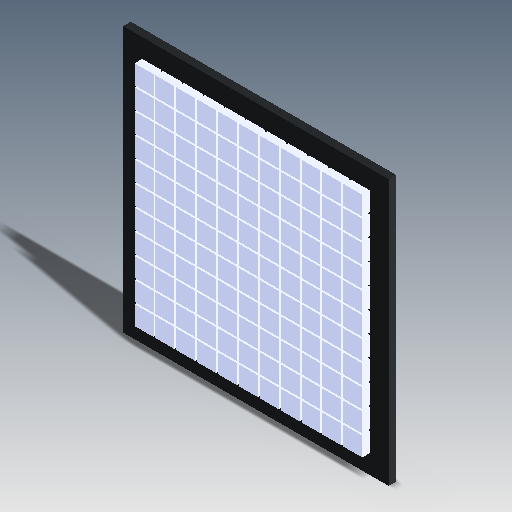
# Autodesk Inventor part: Phase Meter
Saved by Autodesk Inventor 2026 (Build 300175050, 175E)
## iProperties
Created: 2025-08-02
Part Number: Phase Meter
Material: Generic
Document SubType Name: Modeling
Designer: aman0
Density: 1 g/cm^3
Appearance: Default
Author: aman0
Autodesk Inventor part; units mm, degrees
ref_plane "YZ Plane" through (0, 0, 0) normal (1, 0, 0) x (0, 1, 0)
ref_plane "XZ Plane" through (0, 0, 0) normal (0, 1, 0) x (-1, 0, 0)
ref_plane "XY Plane" through (0, 0, 0) normal (0, 0, 1) x (1, 0, 0)
sketch "Sketch1" plane through (0, 0, 0) normal (0, 0, 1) x (1, 0, 0)
  line L0 (-1.25, -1.25) -> (1.25, -1.25)
  line L1 (1.25, -1.25) -> (1.25, 1.25)
  line L2 (1.25, 1.25) -> (-1.25, 1.25)
  line L3 (-1.25, 1.25) -> (-1.25, -1.25)
  line L4 (-1.25, -1.25) -> (1.25, 1.25) construction
  line L5 (1.25, -1.25) -> (-1.25, 1.25) construction
  line L6 (-4, -1.25) -> (-1.5, -1.25)
  line L7 (-1.5, -1.25) -> (-1.5, 1.25)
  line L8 (-1.5, 1.25) -> (-4, 1.25)
  line L9 (-4, 1.25) -> (-4, -1.25)
  line L10 (-4, -1.25) -> (-1.5, 1.25) construction
  line L11 (-1.5, -1.25) -> (-4, 1.25) construction
  line L12 (1.5, -1.25) -> (4, -1.25)
  line L13 (4, -1.25) -> (4, 1.25)
  line L14 (4, 1.25) -> (1.5, 1.25)
  line L15 (1.5, 1.25) -> (1.5, -1.25)
  line L16 (1.5, -1.25) -> (4, 1.25) construction
  line L17 (4, -1.25) -> (1.5, 1.25) construction
  line L18 (-6.75, -1.25) -> (-4.25, -1.25)
  line L19 (-4.25, -1.25) -> (-4.25, 1.25)
  line L20 (-4.25, 1.25) -> (-6.75, 1.25)
  line L21 (-6.75, 1.25) -> (-6.75, -1.25)
  line L22 (-6.75, -1.25) -> (-4.25, 1.25) construction
  line L23 (-4.25, -1.25) -> (-6.75, 1.25) construction
  line L24 (4.25, -1.25) -> (6.75, -1.25)
  line L25 (6.75, -1.25) -> (6.75, 1.25)
  line L26 (6.75, 1.25) -> (4.25, 1.25)
  line L27 (4.25, 1.25) -> (4.25, -1.25)
  line L28 (4.25, -1.25) -> (6.75, 1.25) construction
  line L29 (6.75, -1.25) -> (4.25, 1.25) construction
  line L30 (-9.5, -1.25) -> (-7, -1.25)
  line L31 (-7, -1.25) -> (-7, 1.25)
  line L32 (-7, 1.25) -> (-9.5, 1.25)
  line L33 (-9.5, 1.25) -> (-9.5, -1.25)
  line L34 (-9.5, -1.25) -> (-7, 1.25) construction
  line L35 (-7, -1.25) -> (-9.5, 1.25) construction
  line L36 (7, -1.25) -> (9.5, -1.25)
  line L37 (9.5, -1.25) -> (9.5, 1.25)
  line L38 (9.5, 1.25) -> (7, 1.25)
  line L39 (7, 1.25) -> (7, -1.25)
  line L40 (7, -1.25) -> (9.5, 1.25) construction
  line L41 (9.5, -1.25) -> (7, 1.25) construction
  line L42 (-12.25, -1.25) -> (-9.75, -1.25)
  line L43 (-9.75, -1.25) -> (-9.75, 1.25)
  line L44 (-9.75, 1.25) -> (-12.25, 1.25)
  line L45 (-12.25, 1.25) -> (-12.25, -1.25)
  line L46 (-12.25, -1.25) -> (-9.75, 1.25) construction
  line L47 (-9.75, -1.25) -> (-12.25, 1.25) construction
  line L48 (9.75, -1.25) -> (12.25, -1.25)
  line L49 (12.25, -1.25) -> (12.25, 1.25)
  line L50 (12.25, 1.25) -> (9.75, 1.25)
  line L51 (9.75, 1.25) -> (9.75, -1.25)
  line L52 (9.75, -1.25) -> (12.25, 1.25) construction
  line L53 (12.25, -1.25) -> (9.75, 1.25) construction
  line L54 (-15, -1.25) -> (-12.5, -1.25)
  line L55 (-12.5, -1.25) -> (-12.5, 1.25)
  line L56 (-12.5, 1.25) -> (-15, 1.25)
  line L57 (-15, 1.25) -> (-15, -1.25)
  line L58 (-15, -1.25) -> (-12.5, 1.25) construction
  line L59 (-12.5, -1.25) -> (-15, 1.25) construction
  line L60 (12.5, -1.25) -> (15, -1.25)
  line L61 (15, -1.25) -> (15, 1.25)
  line L62 (15, 1.25) -> (12.5, 1.25)
  line L63 (12.5, 1.25) -> (12.5, -1.25)
  line L64 (12.5, -1.25) -> (15, 1.25) construction
  line L65 (15, -1.25) -> (12.5, 1.25) construction
  line L66 (-1.25, -4) -> (1.25, -4)
  line L67 (1.25, -4) -> (1.25, -1.5)
  line L68 (1.25, -1.5) -> (-1.25, -1.5)
  line L69 (-1.25, -1.5) -> (-1.25, -4)
  line L70 (-1.25, -4) -> (1.25, -1.5) construction
  line L71 (1.25, -4) -> (-1.25, -1.5) construction
  line L72 (-4, -4) -> (-1.5, -4)
  line L73 (-1.5, -4) -> (-1.5, -1.5)
  line L74 (-1.5, -1.5) -> (-4, -1.5)
  line L75 (-4, -1.5) -> (-4, -4)
  line L76 (-4, -4) -> (-1.5, -1.5) construction
  line L77 (-1.5, -4) -> (-4, -1.5) construction
  line L78 (1.5, -4) -> (4, -4)
  line L79 (4, -4) -> (4, -1.5)
  line L80 (4, -1.5) -> (1.5, -1.5)
  line L81 (1.5, -1.5) -> (1.5, -4)
  line L82 (1.5, -4) -> (4, -1.5) construction
  line L83 (4, -4) -> (1.5, -1.5) construction
  line L84 (-6.75, -4) -> (-4.25, -4)
  line L85 (-4.25, -4) -> (-4.25, -1.5)
  line L86 (-4.25, -1.5) -> (-6.75, -1.5)
  line L87 (-6.75, -1.5) -> (-6.75, -4)
  line L88 (-6.75, -4) -> (-4.25, -1.5) construction
  line L89 (-4.25, -4) -> (-6.75, -1.5) construction
  line L90 (4.25, -4) -> (6.75, -4)
  line L91 (6.75, -4) -> (6.75, -1.5)
  line L92 (6.75, -1.5) -> (4.25, -1.5)
  line L93 (4.25, -1.5) -> (4.25, -4)
  line L94 (4.25, -4) -> (6.75, -1.5) construction
  line L95 (6.75, -4) -> (4.25, -1.5) construction
  line L96 (-9.5, -4) -> (-7, -4)
  line L97 (-7, -4) -> (-7, -1.5)
  line L98 (-7, -1.5) -> (-9.5, -1.5)
  line L99 (-9.5, -1.5) -> (-9.5, -4)
  line L100 (-9.5, -4) -> (-7, -1.5) construction
  line L101 (-7, -4) -> (-9.5, -1.5) construction
  line L102 (7, -4) -> (9.5, -4)
  line L103 (9.5, -4) -> (9.5, -1.5)
  line L104 (9.5, -1.5) -> (7, -1.5)
  line L105 (7, -1.5) -> (7, -4)
  line L106 (7, -4) -> (9.5, -1.5) construction
  line L107 (9.5, -4) -> (7, -1.5) construction
  line L108 (-12.25, -4) -> (-9.75, -4)
  line L109 (-9.75, -4) -> (-9.75, -1.5)
  line L110 (-9.75, -1.5) -> (-12.25, -1.5)
  line L111 (-12.25, -1.5) -> (-12.25, -4)
  line L112 (-12.25, -4) -> (-9.75, -1.5) construction
  line L113 (-9.75, -4) -> (-12.25, -1.5) construction
  line L114 (9.75, -4) -> (12.25, -4)
  line L115 (12.25, -4) -> (12.25, -1.5)
  line L116 (12.25, -1.5) -> (9.75, -1.5)
  line L117 (9.75, -1.5) -> (9.75, -4)
  line L118 (9.75, -4) -> (12.25, -1.5) construction
  line L119 (12.25, -4) -> (9.75, -1.5) construction
  line L120 (-15, -4) -> (-12.5, -4)
  line L121 (-12.5, -4) -> (-12.5, -1.5)
  line L122 (-12.5, -1.5) -> (-15, -1.5)
  line L123 (-15, -1.5) -> (-15, -4)
  line L124 (-15, -4) -> (-12.5, -1.5) construction
  line L125 (-12.5, -4) -> (-15, -1.5) construction
  line L126 (12.5, -4) -> (15, -4)
  line L127 (15, -4) -> (15, -1.5)
  line L128 (15, -1.5) -> (12.5, -1.5)
  line L129 (12.5, -1.5) -> (12.5, -4)
  line L130 (12.5, -4) -> (15, -1.5) construction
  line L131 (15, -4) -> (12.5, -1.5) construction
  line L132 (-1.25, 1.5) -> (1.25, 1.5)
  line L133 (1.25, 1.5) -> (1.25, 4)
  line L134 (1.25, 4) -> (-1.25, 4)
  line L135 (-1.25, 4) -> (-1.25, 1.5)
  line L136 (-1.25, 1.5) -> (1.25, 4) construction
  line L137 (1.25, 1.5) -> (-1.25, 4) construction
  line L138 (-4, 1.5) -> (-1.5, 1.5)
  line L139 (-1.5, 1.5) -> (-1.5, 4)
  line L140 (-1.5, 4) -> (-4, 4)
  line L141 (-4, 4) -> (-4, 1.5)
  line L142 (-4, 1.5) -> (-1.5, 4) construction
  line L143 (-1.5, 1.5) -> (-4, 4) construction
  line L144 (1.5, 1.5) -> (4, 1.5)
  line L145 (4, 1.5) -> (4, 4)
  line L146 (4, 4) -> (1.5, 4)
  line L147 (1.5, 4) -> (1.5, 1.5)
  line L148 (1.5, 1.5) -> (4, 4) construction
  line L149 (4, 1.5) -> (1.5, 4) construction
  line L150 (-6.75, 1.5) -> (-4.25, 1.5)
  line L151 (-4.25, 1.5) -> (-4.25, 4)
  line L152 (-4.25, 4) -> (-6.75, 4)
  line L153 (-6.75, 4) -> (-6.75, 1.5)
  line L154 (-6.75, 1.5) -> (-4.25, 4) construction
  line L155 (-4.25, 1.5) -> (-6.75, 4) construction
  line L156 (4.25, 1.5) -> (6.75, 1.5)
  line L157 (6.75, 1.5) -> (6.75, 4)
  line L158 (6.75, 4) -> (4.25, 4)
  line L159 (4.25, 4) -> (4.25, 1.5)
  line L160 (4.25, 1.5) -> (6.75, 4) construction
  line L161 (6.75, 1.5) -> (4.25, 4) construction
  line L162 (-9.5, 1.5) -> (-7, 1.5)
  line L163 (-7, 1.5) -> (-7, 4)
  line L164 (-7, 4) -> (-9.5, 4)
  line L165 (-9.5, 4) -> (-9.5, 1.5)
  line L166 (-9.5, 1.5) -> (-7, 4) construction
  line L167 (-7, 1.5) -> (-9.5, 4) construction
  line L168 (7, 1.5) -> (9.5, 1.5)
  line L169 (9.5, 1.5) -> (9.5, 4)
  line L170 (9.5, 4) -> (7, 4)
  line L171 (7, 4) -> (7, 1.5)
  line L172 (7, 1.5) -> (9.5, 4) construction
  line L173 (9.5, 1.5) -> (7, 4) construction
  line L174 (-12.25, 1.5) -> (-9.75, 1.5)
  line L175 (-9.75, 1.5) -> (-9.75, 4)
  line L176 (-9.75, 4) -> (-12.25, 4)
  line L177 (-12.25, 4) -> (-12.25, 1.5)
  line L178 (-12.25, 1.5) -> (-9.75, 4) construction
  line L179 (-9.75, 1.5) -> (-12.25, 4) construction
  line L180 (9.75, 1.5) -> (12.25, 1.5)
  line L181 (12.25, 1.5) -> (12.25, 4)
  line L182 (12.25, 4) -> (9.75, 4)
  line L183 (9.75, 4) -> (9.75, 1.5)
  line L184 (9.75, 1.5) -> (12.25, 4) construction
  line L185 (12.25, 1.5) -> (9.75, 4) construction
  line L186 (-15, 1.5) -> (-12.5, 1.5)
  line L187 (-12.5, 1.5) -> (-12.5, 4)
  line L188 (-12.5, 4) -> (-15, 4)
  line L189 (-15, 4) -> (-15, 1.5)
  line L190 (-15, 1.5) -> (-12.5, 4) construction
  line L191 (-12.5, 1.5) -> (-15, 4) construction
  line L192 (12.5, 1.5) -> (15, 1.5)
  line L193 (15, 1.5) -> (15, 4)
  line L194 (15, 4) -> (12.5, 4)
  line L195 (12.5, 4) -> (12.5, 1.5)
  line L196 (12.5, 1.5) -> (15, 4) construction
  line L197 (15, 1.5) -> (12.5, 4) construction
  line L198 (-1.25, -6.75) -> (1.25, -6.75)
  line L199 (1.25, -6.75) -> (1.25, -4.25)
  line L200 (1.25, -4.25) -> (-1.25, -4.25)
  line L201 (-1.25, -4.25) -> (-1.25, -6.75)
  line L202 (-1.25, -6.75) -> (1.25, -4.25) construction
  line L203 (1.25, -6.75) -> (-1.25, -4.25) construction
  line L204 (-4, -6.75) -> (-1.5, -6.75)
  line L205 (-1.5, -6.75) -> (-1.5, -4.25)
  line L206 (-1.5, -4.25) -> (-4, -4.25)
  line L207 (-4, -4.25) -> (-4, -6.75)
  line L208 (-4, -6.75) -> (-1.5, -4.25) construction
  line L209 (-1.5, -6.75) -> (-4, -4.25) construction
  line L210 (1.5, -6.75) -> (4, -6.75)
  line L211 (4, -6.75) -> (4, -4.25)
  line L212 (4, -4.25) -> (1.5, -4.25)
  line L213 (1.5, -4.25) -> (1.5, -6.75)
  line L214 (1.5, -6.75) -> (4, -4.25) construction
  line L215 (4, -6.75) -> (1.5, -4.25) construction
  line L216 (-6.75, -6.75) -> (-4.25, -6.75)
  line L217 (-4.25, -6.75) -> (-4.25, -4.25)
  line L218 (-4.25, -4.25) -> (-6.75, -4.25)
  line L219 (-6.75, -4.25) -> (-6.75, -6.75)
  line L220 (-6.75, -6.75) -> (-4.25, -4.25) construction
  line L221 (-4.25, -6.75) -> (-6.75, -4.25) construction
  line L222 (4.25, -6.75) -> (6.75, -6.75)
  line L223 (6.75, -6.75) -> (6.75, -4.25)
  line L224 (6.75, -4.25) -> (4.25, -4.25)
  line L225 (4.25, -4.25) -> (4.25, -6.75)
  line L226 (4.25, -6.75) -> (6.75, -4.25) construction
  line L227 (6.75, -6.75) -> (4.25, -4.25) construction
  line L228 (-9.5, -6.75) -> (-7, -6.75)
  line L229 (-7, -6.75) -> (-7, -4.25)
  line L230 (-7, -4.25) -> (-9.5, -4.25)
  line L231 (-9.5, -4.25) -> (-9.5, -6.75)
  line L232 (-9.5, -6.75) -> (-7, -4.25) construction
  line L233 (-7, -6.75) -> (-9.5, -4.25) construction
  line L234 (7, -6.75) -> (9.5, -6.75)
  line L235 (9.5, -6.75) -> (9.5, -4.25)
  line L236 (9.5, -4.25) -> (7, -4.25)
  line L237 (7, -4.25) -> (7, -6.75)
  line L238 (7, -6.75) -> (9.5, -4.25) construction
  line L239 (9.5, -6.75) -> (7, -4.25) construction
  line L240 (-12.25, -6.75) -> (-9.75, -6.75)
  line L241 (-9.75, -6.75) -> (-9.75, -4.25)
  line L242 (-9.75, -4.25) -> (-12.25, -4.25)
  line L243 (-12.25, -4.25) -> (-12.25, -6.75)
  line L244 (-12.25, -6.75) -> (-9.75, -4.25) construction
  line L245 (-9.75, -6.75) -> (-12.25, -4.25) construction
  line L246 (9.75, -6.75) -> (12.25, -6.75)
  line L247 (12.25, -6.75) -> (12.25, -4.25)
  line L248 (12.25, -4.25) -> (9.75, -4.25)
  line L249 (9.75, -4.25) -> (9.75, -6.75)
  line L250 (9.75, -6.75) -> (12.25, -4.25) construction
  line L251 (12.25, -6.75) -> (9.75, -4.25) construction
  line L252 (-15, -6.75) -> (-12.5, -6.75)
  line L253 (-12.5, -6.75) -> (-12.5, -4.25)
  line L254 (-12.5, -4.25) -> (-15, -4.25)
  line L255 (-15, -4.25) -> (-15, -6.75)
  line L256 (-15, -6.75) -> (-12.5, -4.25) construction
  line L257 (-12.5, -6.75) -> (-15, -4.25) construction
  line L258 (12.5, -6.75) -> (15, -6.75)
  line L259 (15, -6.75) -> (15, -4.25)
  line L260 (15, -4.25) -> (12.5, -4.25)
  line L261 (12.5, -4.25) -> (12.5, -6.75)
  line L262 (12.5, -6.75) -> (15, -4.25) construction
  line L263 (15, -6.75) -> (12.5, -4.25) construction
  line L264 (-1.25, 4.25) -> (1.25, 4.25)
  line L265 (1.25, 4.25) -> (1.25, 6.75)
  line L266 (1.25, 6.75) -> (-1.25, 6.75)
  line L267 (-1.25, 6.75) -> (-1.25, 4.25)
  line L268 (-1.25, 4.25) -> (1.25, 6.75) construction
  line L269 (1.25, 4.25) -> (-1.25, 6.75) construction
  line L270 (-4, 4.25) -> (-1.5, 4.25)
  line L271 (-1.5, 4.25) -> (-1.5, 6.75)
  line L272 (-1.5, 6.75) -> (-4, 6.75)
  line L273 (-4, 6.75) -> (-4, 4.25)
  line L274 (-4, 4.25) -> (-1.5, 6.75) construction
  line L275 (-1.5, 4.25) -> (-4, 6.75) construction
  line L276 (1.5, 4.25) -> (4, 4.25)
  line L277 (4, 4.25) -> (4, 6.75)
  line L278 (4, 6.75) -> (1.5, 6.75)
  line L279 (1.5, 6.75) -> (1.5, 4.25)
  line L280 (1.5, 4.25) -> (4, 6.75) construction
  line L281 (4, 4.25) -> (1.5, 6.75) construction
  line L282 (-6.75, 4.25) -> (-4.25, 4.25)
  line L283 (-4.25, 4.25) -> (-4.25, 6.75)
  line L284 (-4.25, 6.75) -> (-6.75, 6.75)
  line L285 (-6.75, 6.75) -> (-6.75, 4.25)
  line L286 (-6.75, 4.25) -> (-4.25, 6.75) construction
  line L287 (-4.25, 4.25) -> (-6.75, 6.75) construction
  line L288 (4.25, 4.25) -> (6.75, 4.25)
  line L289 (6.75, 4.25) -> (6.75, 6.75)
  line L290 (6.75, 6.75) -> (4.25, 6.75)
  line L291 (4.25, 6.75) -> (4.25, 4.25)
  line L292 (4.25, 4.25) -> (6.75, 6.75) construction
  line L293 (6.75, 4.25) -> (4.25, 6.75) construction
  line L294 (-9.5, 4.25) -> (-7, 4.25)
  line L295 (-7, 4.25) -> (-7, 6.75)
  line L296 (-7, 6.75) -> (-9.5, 6.75)
  line L297 (-9.5, 6.75) -> (-9.5, 4.25)
  line L298 (-9.5, 4.25) -> (-7, 6.75) construction
  line L299 (-7, 4.25) -> (-9.5, 6.75) construction
  line L300 (7, 4.25) -> (9.5, 4.25)
  line L301 (9.5, 4.25) -> (9.5, 6.75)
  line L302 (9.5, 6.75) -> (7, 6.75)
  line L303 (7, 6.75) -> (7, 4.25)
  line L304 (7, 4.25) -> (9.5, 6.75) construction
  line L305 (9.5, 4.25) -> (7, 6.75) construction
  line L306 (-12.25, 4.25) -> (-9.75, 4.25)
  line L307 (-9.75, 4.25) -> (-9.75, 6.75)
  line L308 (-9.75, 6.75) -> (-12.25, 6.75)
  line L309 (-12.25, 6.75) -> (-12.25, 4.25)
  line L310 (-12.25, 4.25) -> (-9.75, 6.75) construction
  line L311 (-9.75, 4.25) -> (-12.25, 6.75) construction
  line L312 (9.75, 4.25) -> (12.25, 4.25)
  line L313 (12.25, 4.25) -> (12.25, 6.75)
  line L314 (12.25, 6.75) -> (9.75, 6.75)
  line L315 (9.75, 6.75) -> (9.75, 4.25)
  line L316 (9.75, 4.25) -> (12.25, 6.75) construction
  line L317 (12.25, 4.25) -> (9.75, 6.75) construction
  line L318 (-15, 4.25) -> (-12.5, 4.25)
  line L319 (-12.5, 4.25) -> (-12.5, 6.75)
  line L320 (-12.5, 6.75) -> (-15, 6.75)
  line L321 (-15, 6.75) -> (-15, 4.25)
  line L322 (-15, 4.25) -> (-12.5, 6.75) construction
  line L323 (-12.5, 4.25) -> (-15, 6.75) construction
  line L324 (12.5, 4.25) -> (15, 4.25)
  line L325 (15, 4.25) -> (15, 6.75)
  line L326 (15, 6.75) -> (12.5, 6.75)
  line L327 (12.5, 6.75) -> (12.5, 4.25)
  line L328 (12.5, 4.25) -> (15, 6.75) construction
  line L329 (15, 4.25) -> (12.5, 6.75) construction
  line L330 (-1.25, -9.5) -> (1.25, -9.5)
  line L331 (1.25, -9.5) -> (1.25, -7)
  line L332 (1.25, -7) -> (-1.25, -7)
  line L333 (-1.25, -7) -> (-1.25, -9.5)
  line L334 (-1.25, -9.5) -> (1.25, -7) construction
  line L335 (1.25, -9.5) -> (-1.25, -7) construction
  line L336 (-4, -9.5) -> (-1.5, -9.5)
  line L337 (-1.5, -9.5) -> (-1.5, -7)
  line L338 (-1.5, -7) -> (-4, -7)
  line L339 (-4, -7) -> (-4, -9.5)
  line L340 (-4, -9.5) -> (-1.5, -7) construction
  line L341 (-1.5, -9.5) -> (-4, -7) construction
  line L342 (1.5, -9.5) -> (4, -9.5)
  line L343 (4, -9.5) -> (4, -7)
  line L344 (4, -7) -> (1.5, -7)
  line L345 (1.5, -7) -> (1.5, -9.5)
  line L346 (1.5, -9.5) -> (4, -7) construction
  line L347 (4, -9.5) -> (1.5, -7) construction
  line L348 (-6.75, -9.5) -> (-4.25, -9.5)
  line L349 (-4.25, -9.5) -> (-4.25, -7)
  line L350 (-4.25, -7) -> (-6.75, -7)
  line L351 (-6.75, -7) -> (-6.75, -9.5)
  line L352 (-6.75, -9.5) -> (-4.25, -7) construction
  line L353 (-4.25, -9.5) -> (-6.75, -7) construction
  line L354 (4.25, -9.5) -> (6.75, -9.5)
  line L355 (6.75, -9.5) -> (6.75, -7)
  line L356 (6.75, -7) -> (4.25, -7)
  line L357 (4.25, -7) -> (4.25, -9.5)
  line L358 (4.25, -9.5) -> (6.75, -7) construction
  line L359 (6.75, -9.5) -> (4.25, -7) construction
  line L360 (-9.5, -9.5) -> (-7, -9.5)
  line L361 (-7, -9.5) -> (-7, -7)
  line L362 (-7, -7) -> (-9.5, -7)
  line L363 (-9.5, -7) -> (-9.5, -9.5)
  line L364 (-9.5, -9.5) -> (-7, -7) construction
  line L365 (-7, -9.5) -> (-9.5, -7) construction
  line L366 (7, -9.5) -> (9.5, -9.5)
  line L367 (9.5, -9.5) -> (9.5, -7)
  line L368 (9.5, -7) -> (7, -7)
  line L369 (7, -7) -> (7, -9.5)
  line L370 (7, -9.5) -> (9.5, -7) construction
  line L371 (9.5, -9.5) -> (7, -7) construction
  line L372 (-12.25, -9.5) -> (-9.75, -9.5)
  line L373 (-9.75, -9.5) -> (-9.75, -7)
  line L374 (-9.75, -7) -> (-12.25, -7)
  line L375 (-12.25, -7) -> (-12.25, -9.5)
  line L376 (-12.25, -9.5) -> (-9.75, -7) construction
  line L377 (-9.75, -9.5) -> (-12.25, -7) construction
  line L378 (9.75, -9.5) -> (12.25, -9.5)
  line L379 (12.25, -9.5) -> (12.25, -7)
  line L380 (12.25, -7) -> (9.75, -7)
  line L381 (9.75, -7) -> (9.75, -9.5)
  line L382 (9.75, -9.5) -> (12.25, -7) construction
  line L383 (12.25, -9.5) -> (9.75, -7) construction
  line L384 (-15, -9.5) -> (-12.5, -9.5)
  line L385 (-12.5, -9.5) -> (-12.5, -7)
  line L386 (-12.5, -7) -> (-15, -7)
  line L387 (-15, -7) -> (-15, -9.5)
  line L388 (-15, -9.5) -> (-12.5, -7) construction
  line L389 (-12.5, -9.5) -> (-15, -7) construction
  line L390 (12.5, -9.5) -> (15, -9.5)
  line L391 (15, -9.5) -> (15, -7)
  line L392 (15, -7) -> (12.5, -7)
  line L393 (12.5, -7) -> (12.5, -9.5)
  line L394 (12.5, -9.5) -> (15, -7) construction
  line L395 (15, -9.5) -> (12.5, -7) construction
  line L396 (-1.25, 7) -> (1.25, 7)
  line L397 (1.25, 7) -> (1.25, 9.5)
  line L398 (1.25, 9.5) -> (-1.25, 9.5)
  line L399 (-1.25, 9.5) -> (-1.25, 7)
  line L400 (-1.25, 7) -> (1.25, 9.5) construction
  line L401 (1.25, 7) -> (-1.25, 9.5) construction
  line L402 (-4, 7) -> (-1.5, 7)
  line L403 (-1.5, 7) -> (-1.5, 9.5)
  line L404 (-1.5, 9.5) -> (-4, 9.5)
  line L405 (-4, 9.5) -> (-4, 7)
  line L406 (-4, 7) -> (-1.5, 9.5) construction
  line L407 (-1.5, 7) -> (-4, 9.5) construction
  line L408 (1.5, 7) -> (4, 7)
  line L409 (4, 7) -> (4, 9.5)
  line L410 (4, 9.5) -> (1.5, 9.5)
  line L411 (1.5, 9.5) -> (1.5, 7)
  line L412 (1.5, 7) -> (4, 9.5) construction
  line L413 (4, 7) -> (1.5, 9.5) construction
  line L414 (-6.75, 7) -> (-4.25, 7)
  line L415 (-4.25, 7) -> (-4.25, 9.5)
  line L416 (-4.25, 9.5) -> (-6.75, 9.5)
  line L417 (-6.75, 9.5) -> (-6.75, 7)
  line L418 (-6.75, 7) -> (-4.25, 9.5) construction
  line L419 (-4.25, 7) -> (-6.75, 9.5) construction
  line L420 (4.25, 7) -> (6.75, 7)
  line L421 (6.75, 7) -> (6.75, 9.5)
  line L422 (6.75, 9.5) -> (4.25, 9.5)
  line L423 (4.25, 9.5) -> (4.25, 7)
  line L424 (4.25, 7) -> (6.75, 9.5) construction
  line L425 (6.75, 7) -> (4.25, 9.5) construction
  line L426 (-9.5, 7) -> (-7, 7)
  line L427 (-7, 7) -> (-7, 9.5)
  line L428 (-7, 9.5) -> (-9.5, 9.5)
  line L429 (-9.5, 9.5) -> (-9.5, 7)
  line L430 (-9.5, 7) -> (-7, 9.5) construction
  line L431 (-7, 7) -> (-9.5, 9.5) construction
  line L432 (7, 7) -> (9.5, 7)
  line L433 (9.5, 7) -> (9.5, 9.5)
  line L434 (9.5, 9.5) -> (7, 9.5)
  line L435 (7, 9.5) -> (7, 7)
  line L436 (7, 7) -> (9.5, 9.5) construction
  line L437 (9.5, 7) -> (7, 9.5) construction
  line L438 (-12.25, 7) -> (-9.75, 7)
  line L439 (-9.75, 7) -> (-9.75, 9.5)
  line L440 (-9.75, 9.5) -> (-12.25, 9.5)
  line L441 (-12.25, 9.5) -> (-12.25, 7)
  line L442 (-12.25, 7) -> (-9.75, 9.5) construction
  line L443 (-9.75, 7) -> (-12.25, 9.5) construction
  line L444 (9.75, 7) -> (12.25, 7)
  line L445 (12.25, 7) -> (12.25, 9.5)
  line L446 (12.25, 9.5) -> (9.75, 9.5)
  line L447 (9.75, 9.5) -> (9.75, 7)
  line L448 (9.75, 7) -> (12.25, 9.5) construction
  line L449 (12.25, 7) -> (9.75, 9.5) construction
  line L450 (-15, 7) -> (-12.5, 7)
  line L451 (-12.5, 7) -> (-12.5, 9.5)
  line L452 (-12.5, 9.5) -> (-15, 9.5)
  line L453 (-15, 9.5) -> (-15, 7)
  line L454 (-15, 7) -> (-12.5, 9.5) construction
  line L455 (-12.5, 7) -> (-15, 9.5) construction
  line L456 (12.5, 7) -> (15, 7)
  line L457 (15, 7) -> (15, 9.5)
  line L458 (15, 9.5) -> (12.5, 9.5)
  line L459 (12.5, 9.5) -> (12.5, 7)
  line L460 (12.5, 7) -> (15, 9.5) construction
  line L461 (15, 7) -> (12.5, 9.5) construction
  line L462 (-1.25, -12.25) -> (1.25, -12.25)
  line L463 (1.25, -12.25) -> (1.25, -9.75)
  line L464 (1.25, -9.75) -> (-1.25, -9.75)
  line L465 (-1.25, -9.75) -> (-1.25, -12.25)
  line L466 (-1.25, -12.25) -> (1.25, -9.75) construction
  line L467 (1.25, -12.25) -> (-1.25, -9.75) construction
  line L468 (-4, -12.25) -> (-1.5, -12.25)
  line L469 (-1.5, -12.25) -> (-1.5, -9.75)
  line L470 (-1.5, -9.75) -> (-4, -9.75)
  line L471 (-4, -9.75) -> (-4, -12.25)
  line L472 (-4, -12.25) -> (-1.5, -9.75) construction
  line L473 (-1.5, -12.25) -> (-4, -9.75) construction
  line L474 (1.5, -12.25) -> (4, -12.25)
  line L475 (4, -12.25) -> (4, -9.75)
  line L476 (4, -9.75) -> (1.5, -9.75)
  line L477 (1.5, -9.75) -> (1.5, -12.25)
  line L478 (1.5, -12.25) -> (4, -9.75) construction
  line L479 (4, -12.25) -> (1.5, -9.75) construction
  line L480 (-6.75, -12.25) -> (-4.25, -12.25)
  line L481 (-4.25, -12.25) -> (-4.25, -9.75)
  line L482 (-4.25, -9.75) -> (-6.75, -9.75)
  line L483 (-6.75, -9.75) -> (-6.75, -12.25)
  line L484 (-6.75, -12.25) -> (-4.25, -9.75) construction
  line L485 (-4.25, -12.25) -> (-6.75, -9.75) construction
  line L486 (4.25, -12.25) -> (6.75, -12.25)
  line L487 (6.75, -12.25) -> (6.75, -9.75)
  line L488 (6.75, -9.75) -> (4.25, -9.75)
  line L489 (4.25, -9.75) -> (4.25, -12.25)
  line L490 (4.25, -12.25) -> (6.75, -9.75) construction
  line L491 (6.75, -12.25) -> (4.25, -9.75) construction
  line L492 (-9.5, -12.25) -> (-7, -12.25)
  line L493 (-7, -12.25) -> (-7, -9.75)
  line L494 (-7, -9.75) -> (-9.5, -9.75)
  line L495 (-9.5, -9.75) -> (-9.5, -12.25)
  line L496 (-9.5, -12.25) -> (-7, -9.75) construction
  line L497 (-7, -12.25) -> (-9.5, -9.75) construction
  line L498 (7, -12.25) -> (9.5, -12.25)
  line L499 (9.5, -12.25) -> (9.5, -9.75)
  line L500 (9.5, -9.75) -> (7, -9.75)
  line L501 (7, -9.75) -> (7, -12.25)
  line L502 (7, -12.25) -> (9.5, -9.75) construction
  line L503 (9.5, -12.25) -> (7, -9.75) construction
  line L504 (-12.25, -12.25) -> (-9.75, -12.25)
  line L505 (-9.75, -12.25) -> (-9.75, -9.75)
  line L506 (-9.75, -9.75) -> (-12.25, -9.75)
  line L507 (-12.25, -9.75) -> (-12.25, -12.25)
  line L508 (-12.25, -12.25) -> (-9.75, -9.75) construction
  line L509 (-9.75, -12.25) -> (-12.25, -9.75) construction
  line L510 (9.75, -12.25) -> (12.25, -12.25)
  line L511 (12.25, -12.25) -> (12.25, -9.75)
  line L512 (12.25, -9.75) -> (9.75, -9.75)
  line L513 (9.75, -9.75) -> (9.75, -12.25)
  line L514 (9.75, -12.25) -> (12.25, -9.75) construction
  line L515 (12.25, -12.25) -> (9.75, -9.75) construction
  line L516 (-15, -12.25) -> (-12.5, -12.25)
  line L517 (-12.5, -12.25) -> (-12.5, -9.75)
  line L518 (-12.5, -9.75) -> (-15, -9.75)
  line L519 (-15, -9.75) -> (-15, -12.25)
  line L520 (-15, -12.25) -> (-12.5, -9.75) construction
  line L521 (-12.5, -12.25) -> (-15, -9.75) construction
  line L522 (12.5, -12.25) -> (15, -12.25)
  line L523 (15, -12.25) -> (15, -9.75)
  line L524 (15, -9.75) -> (12.5, -9.75)
  line L525 (12.5, -9.75) -> (12.5, -12.25)
  line L526 (12.5, -12.25) -> (15, -9.75) construction
  line L527 (15, -12.25) -> (12.5, -9.75) construction
  line L528 (-1.25, 9.75) -> (1.25, 9.75)
  line L529 (1.25, 9.75) -> (1.25, 12.25)
  line L530 (1.25, 12.25) -> (-1.25, 12.25)
  line L531 (-1.25, 12.25) -> (-1.25, 9.75)
  line L532 (-1.25, 9.75) -> (1.25, 12.25) construction
  line L533 (1.25, 9.75) -> (-1.25, 12.25) construction
  line L534 (-4, 9.75) -> (-1.5, 9.75)
  line L535 (-1.5, 9.75) -> (-1.5, 12.25)
  line L536 (-1.5, 12.25) -> (-4, 12.25)
  line L537 (-4, 12.25) -> (-4, 9.75)
  line L538 (-4, 9.75) -> (-1.5, 12.25) construction
  line L539 (-1.5, 9.75) -> (-4, 12.25) construction
  line L540 (1.5, 9.75) -> (4, 9.75)
  line L541 (4, 9.75) -> (4, 12.25)
  line L542 (4, 12.25) -> (1.5, 12.25)
  line L543 (1.5, 12.25) -> (1.5, 9.75)
  line L544 (1.5, 9.75) -> (4, 12.25) construction
  line L545 (4, 9.75) -> (1.5, 12.25) construction
  line L546 (-6.75, 9.75) -> (-4.25, 9.75)
  line L547 (-4.25, 9.75) -> (-4.25, 12.25)
  line L548 (-4.25, 12.25) -> (-6.75, 12.25)
  line L549 (-6.75, 12.25) -> (-6.75, 9.75)
  line L550 (-6.75, 9.75) -> (-4.25, 12.25) construction
  line L551 (-4.25, 9.75) -> (-6.75, 12.25) construction
  line L552 (4.25, 9.75) -> (6.75, 9.75)
  line L553 (6.75, 9.75) -> (6.75, 12.25)
  line L554 (6.75, 12.25) -> (4.25, 12.25)
  line L555 (4.25, 12.25) -> (4.25, 9.75)
  line L556 (4.25, 9.75) -> (6.75, 12.25) construction
  line L557 (6.75, 9.75) -> (4.25, 12.25) construction
  line L558 (-9.5, 9.75) -> (-7, 9.75)
  line L559 (-7, 9.75) -> (-7, 12.25)
  line L560 (-7, 12.25) -> (-9.5, 12.25)
  line L561 (-9.5, 12.25) -> (-9.5, 9.75)
  line L562 (-9.5, 9.75) -> (-7, 12.25) construction
  line L563 (-7, 9.75) -> (-9.5, 12.25) construction
  line L564 (7, 9.75) -> (9.5, 9.75)
  line L565 (9.5, 9.75) -> (9.5, 12.25)
  line L566 (9.5, 12.25) -> (7, 12.25)
  line L567 (7, 12.25) -> (7, 9.75)
  line L568 (7, 9.75) -> (9.5, 12.25) construction
  line L569 (9.5, 9.75) -> (7, 12.25) construction
  line L570 (-12.25, 9.75) -> (-9.75, 9.75)
  line L571 (-9.75, 9.75) -> (-9.75, 12.25)
  line L572 (-9.75, 12.25) -> (-12.25, 12.25)
  line L573 (-12.25, 12.25) -> (-12.25, 9.75)
  line L574 (-12.25, 9.75) -> (-9.75, 12.25) construction
  line L575 (-9.75, 9.75) -> (-12.25, 12.25) construction
  line L576 (9.75, 9.75) -> (12.25, 9.75)
  line L577 (12.25, 9.75) -> (12.25, 12.25)
  line L578 (12.25, 12.25) -> (9.75, 12.25)
  line L579 (9.75, 12.25) -> (9.75, 9.75)
  line L580 (9.75, 9.75) -> (12.25, 12.25) construction
  line L581 (12.25, 9.75) -> (9.75, 12.25) construction
  line L582 (-15, 9.75) -> (-12.5, 9.75)
  line L583 (-12.5, 9.75) -> (-12.5, 12.25)
  line L584 (-12.5, 12.25) -> (-15, 12.25)
  line L585 (-15, 12.25) -> (-15, 9.75)
  line L586 (-15, 9.75) -> (-12.5, 12.25) construction
  line L587 (-12.5, 9.75) -> (-15, 12.25) construction
  line L588 (12.5, 9.75) -> (15, 9.75)
  line L589 (15, 9.75) -> (15, 12.25)
  line L590 (15, 12.25) -> (12.5, 12.25)
  line L591 (12.5, 12.25) -> (12.5, 9.75)
  line L592 (12.5, 9.75) -> (15, 12.25) construction
  line L593 (15, 9.75) -> (12.5, 12.25) construction
  line L594 (-1.25, -15) -> (1.25, -15)
  line L595 (1.25, -15) -> (1.25, -12.5)
  line L596 (1.25, -12.5) -> (-1.25, -12.5)
  line L597 (-1.25, -12.5) -> (-1.25, -15)
  line L598 (-1.25, -15) -> (1.25, -12.5) construction
  line L599 (1.25, -15) -> (-1.25, -12.5) construction
  line L600 (-4, -15) -> (-1.5, -15)
  line L601 (-1.5, -15) -> (-1.5, -12.5)
  line L602 (-1.5, -12.5) -> (-4, -12.5)
  line L603 (-4, -12.5) -> (-4, -15)
  line L604 (-4, -15) -> (-1.5, -12.5) construction
  line L605 (-1.5, -15) -> (-4, -12.5) construction
  line L606 (1.5, -15) -> (4, -15)
  line L607 (4, -15) -> (4, -12.5)
  line L608 (4, -12.5) -> (1.5, -12.5)
  line L609 (1.5, -12.5) -> (1.5, -15)
  line L610 (1.5, -15) -> (4, -12.5) construction
  line L611 (4, -15) -> (1.5, -12.5) construction
  line L612 (-6.75, -15) -> (-4.25, -15)
  line L613 (-4.25, -15) -> (-4.25, -12.5)
  line L614 (-4.25, -12.5) -> (-6.75, -12.5)
  line L615 (-6.75, -12.5) -> (-6.75, -15)
  line L616 (-6.75, -15) -> (-4.25, -12.5) construction
  line L617 (-4.25, -15) -> (-6.75, -12.5) construction
  line L618 (4.25, -15) -> (6.75, -15)
  line L619 (6.75, -15) -> (6.75, -12.5)
  line L620 (6.75, -12.5) -> (4.25, -12.5)
  line L621 (4.25, -12.5) -> (4.25, -15)
  line L622 (4.25, -15) -> (6.75, -12.5) construction
  line L623 (6.75, -15) -> (4.25, -12.5) construction
  line L624 (-9.5, -15) -> (-7, -15)
  line L625 (-7, -15) -> (-7, -12.5)
  line L626 (-7, -12.5) -> (-9.5, -12.5)
  line L627 (-9.5, -12.5) -> (-9.5, -15)
  line L628 (-9.5, -15) -> (-7, -12.5) construction
  line L629 (-7, -15) -> (-9.5, -12.5) construction
  line L630 (7, -15) -> (9.5, -15)
  line L631 (9.5, -15) -> (9.5, -12.5)
  line L632 (9.5, -12.5) -> (7, -12.5)
  line L633 (7, -12.5) -> (7, -15)
  line L634 (7, -15) -> (9.5, -12.5) construction
  line L635 (9.5, -15) -> (7, -12.5) construction
  line L636 (-12.25, -15) -> (-9.75, -15)
  line L637 (-9.75, -15) -> (-9.75, -12.5)
  line L638 (-9.75, -12.5) -> (-12.25, -12.5)
  line L639 (-12.25, -12.5) -> (-12.25, -15)
  line L640 (-12.25, -15) -> (-9.75, -12.5) construction
  line L641 (-9.75, -15) -> (-12.25, -12.5) construction
  line L642 (9.75, -15) -> (12.25, -15)
  line L643 (12.25, -15) -> (12.25, -12.5)
  line L644 (12.25, -12.5) -> (9.75, -12.5)
  line L645 (9.75, -12.5) -> (9.75, -15)
  line L646 (9.75, -15) -> (12.25, -12.5) construction
  line L647 (12.25, -15) -> (9.75, -12.5) construction
  line L648 (-15, -15) -> (-12.5, -15)
  line L649 (-12.5, -15) -> (-12.5, -12.5)
  line L650 (-12.5, -12.5) -> (-15, -12.5)
  line L651 (-15, -12.5) -> (-15, -15)
  line L652 (-15, -15) -> (-12.5, -12.5) construction
  line L653 (-12.5, -15) -> (-15, -12.5) construction
  line L654 (12.5, -15) -> (15, -15)
  line L655 (15, -15) -> (15, -12.5)
  line L656 (15, -12.5) -> (12.5, -12.5)
  line L657 (12.5, -12.5) -> (12.5, -15)
  line L658 (12.5, -15) -> (15, -12.5) construction
  line L659 (15, -15) -> (12.5, -12.5) construction
  line L660 (-1.25, 12.5) -> (1.25, 12.5)
  line L661 (1.25, 12.5) -> (1.25, 15)
  line L662 (1.25, 15) -> (-1.25, 15)
  line L663 (-1.25, 15) -> (-1.25, 12.5)
  line L664 (-1.25, 12.5) -> (1.25, 15) construction
  line L665 (1.25, 12.5) -> (-1.25, 15) construction
  line L666 (-4, 12.5) -> (-1.5, 12.5)
  line L667 (-1.5, 12.5) -> (-1.5, 15)
  line L668 (-1.5, 15) -> (-4, 15)
  line L669 (-4, 15) -> (-4, 12.5)
  line L670 (-4, 12.5) -> (-1.5, 15) construction
  line L671 (-1.5, 12.5) -> (-4, 15) construction
  line L672 (1.5, 12.5) -> (4, 12.5)
  line L673 (4, 12.5) -> (4, 15)
  line L674 (4, 15) -> (1.5, 15)
  line L675 (1.5, 15) -> (1.5, 12.5)
  line L676 (1.5, 12.5) -> (4, 15) construction
  line L677 (4, 12.5) -> (1.5, 15) construction
  line L678 (-6.75, 12.5) -> (-4.25, 12.5)
  line L679 (-4.25, 12.5) -> (-4.25, 15)
  line L680 (-4.25, 15) -> (-6.75, 15)
  line L681 (-6.75, 15) -> (-6.75, 12.5)
  line L682 (-6.75, 12.5) -> (-4.25, 15) construction
  line L683 (-4.25, 12.5) -> (-6.75, 15) construction
  line L684 (4.25, 12.5) -> (6.75, 12.5)
  line L685 (6.75, 12.5) -> (6.75, 15)
  line L686 (6.75, 15) -> (4.25, 15)
  line L687 (4.25, 15) -> (4.25, 12.5)
  line L688 (4.25, 12.5) -> (6.75, 15) construction
  line L689 (6.75, 12.5) -> (4.25, 15) construction
  line L690 (-9.5, 12.5) -> (-7, 12.5)
  line L691 (-7, 12.5) -> (-7, 15)
  line L692 (-7, 15) -> (-9.5, 15)
  line L693 (-9.5, 15) -> (-9.5, 12.5)
  line L694 (-9.5, 12.5) -> (-7, 15) construction
  line L695 (-7, 12.5) -> (-9.5, 15) construction
  line L696 (7, 12.5) -> (9.5, 12.5)
  line L697 (9.5, 12.5) -> (9.5, 15)
  line L698 (9.5, 15) -> (7, 15)
  line L699 (7, 15) -> (7, 12.5)
  line L700 (7, 12.5) -> (9.5, 15) construction
  line L701 (9.5, 12.5) -> (7, 15) construction
  line L702 (-12.25, 12.5) -> (-9.75, 12.5)
  line L703 (-9.75, 12.5) -> (-9.75, 15)
  line L704 (-9.75, 15) -> (-12.25, 15)
  line L705 (-12.25, 15) -> (-12.25, 12.5)
  line L706 (-12.25, 12.5) -> (-9.75, 15) construction
  line L707 (-9.75, 12.5) -> (-12.25, 15) construction
  line L708 (9.75, 12.5) -> (12.25, 12.5)
  line L709 (12.25, 12.5) -> (12.25, 15)
  line L710 (12.25, 15) -> (9.75, 15)
  line L711 (9.75, 15) -> (9.75, 12.5)
  line L712 (9.75, 12.5) -> (12.25, 15) construction
  line L713 (12.25, 12.5) -> (9.75, 15) construction
  line L714 (-15, 12.5) -> (-12.5, 12.5)
  line L715 (-12.5, 12.5) -> (-12.5, 15)
  line L716 (-12.5, 15) -> (-15, 15)
  line L717 (-15, 15) -> (-15, 12.5)
  line L718 (-15, 12.5) -> (-12.5, 15) construction
  line L719 (-12.5, 12.5) -> (-15, 15) construction
  line L720 (12.5, 12.5) -> (15, 12.5)
  line L721 (15, 12.5) -> (15, 15)
  line L722 (15, 15) -> (12.5, 15)
  line L723 (12.5, 15) -> (12.5, 12.5)
  line L724 (12.5, 12.5) -> (15, 15) construction
  line L725 (15, 12.5) -> (12.5, 15) construction
  point P0 (0, 0)
  dimension "d0" = 2.5
  dimension "d1" = 2.5
  dimension "d4" = 2.75
  dimension "d7" = 2.75
  constraints: 1452 end point, 2 collinear, 2 horizontal, 2 midpoint, 2 parallel, 1 perpendicular, 1 vertical, 1198 other
  measures "d0" distance of L0.start L0.end
  measures "d1" distance of L1.end L0.end
  measures "d4" distance of L0.start L6.start
  measures "d7" distance of L0.start L66.start
extrude "Extrusion1" add sketch "Sketch1" along normal blind 1
sketch "Sketch2" plane through (0, 0, 0) normal (0, 0, -1) x (-1, 0, 0)
  line L0 (-17.5, -17.5) -> (17.5, -17.5)
  line L1 (17.5, -17.5) -> (17.5, 17.5)
  line L2 (17.5, 17.5) -> (-17.5, 17.5)
  line L3 (-17.5, 17.5) -> (-17.5, -17.5)
  line L4 (-17.5, -17.5) -> (17.5, 17.5) construction
  line L5 (17.5, -17.5) -> (-17.5, 17.5) construction
  point P0 (0, 0)
  dimension "d12" = 35
  dimension "d13" = 35
  constraints: 12 end point, 2 midpoint, 2 parallel, 1 horizontal, 1 perpendicular
  measures "d12" distance of L0.start L0.end
  measures "d13" distance of L1.end L0.end
extrude "Extrusion2" add sketch "Sketch2" along normal blind 1
body "Solid1"
